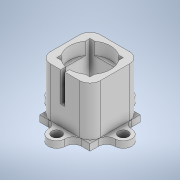
# Autodesk Inventor part: SpringPotBottom
Saved by Autodesk Inventor 2022 (Build 260153000, 153)
## iProperties
Created: 2022-04-06
Part Number: SpringPotBottom
Material: Generic
Document SubType Name: Modeling
Designer: awp
Density: 1 g/cm^3
Appearance: Default
Author: awp
Autodesk Inventor part; units mm, degrees
ref_plane "YZ Plane" through (0, 0, 0) normal (1, 0, 0) x (0, 1, 0)
ref_plane "XZ Plane" through (0, 0, 0) normal (0, 1, 0) x (-1, 0, 0)
ref_plane "XY Plane" through (0, 0, 0) normal (0, 0, 1) x (1, 0, 0)
sketch "Sketch1" plane through (0, 0, 0) normal (0, 1, 0) x (-1, 0, 0)
  line L0 (0, 0) -> (10.125, 0)
  line L1 (10.125, 0) -> (10.125, -10.125)
  line L2 (10.125, -10.125) -> (0, -10.125)
  line L3 (0, -10.125) -> (0, 0)
  line L4 (10.125, -10.125) -> (12.665, -10.125)
  line L5 (12.665, -10.125) -> (12.665, -12.665)
  line L6 (12.665, -12.665) -> (10.125, -12.665)
  line L7 (10.125, -12.665) -> (10.125, -10.125)
  line L8 (0, 0) -> (-2.54, 0)
  line L9 (-2.54, 0) -> (-2.54, 2.54)
  line L10 (-2.54, 2.54) -> (0, 2.54)
  line L11 (0, 2.54) -> (0, 0)
  line L12 (-2.54, 2.54) -> (12.665, 2.54)
  line L13 (12.665, 2.54) -> (12.665, -12.665)
  line L14 (12.665, -12.665) -> (-2.54, -12.665)
  line L15 (-2.54, -12.665) -> (-2.54, 2.54)
  dimension "d0" = 10.125
  dimension "d1" = 10.125
  dimension "d2" = 2.54
  dimension "d3" = 2.54
  dimension "d4" = 2.54
  dimension "d5" = 2.54
  constraints: 32 end point, 8 parallel, 4 horizontal, 4 perpendicular
  measures "d0" distance of L1.end L2.end
  measures "d1" distance of L0.end L1.end
  measures "d2" distance of L5.end L6.end
  measures "d3" distance of L4.end L5.end
  measures "d4" distance of L9.end L10.end
  measures "d5" distance of L8.end L9.end
extrude "Extrusion1" add sketch "Sketch1" along normal blind 8 contours L11 L12 L13 L4 L1 L0 | L3 L2 L7 L14 L15 L8 | L8 L9 L10 L11 | L4 L5 L6 L7
sketch "Sketch2" plane through (0, 8, 0) normal (0, 1, 0) x (1, 0, 0)
  line L0 (2.54, -2.54) -> (-5.0625, -2.54)
  line L1 (-12.665, -2.54) -> (2.54, -2.54) projected
  line L2 (-5.0625, -2.54) -> (-5.0625, 0)
  line L3 (0, 0) -> (-10.125, 0) projected
  line L4 (-5.0625, -2.54) -> (-6.3325, -2.54)
  line L5 (-6.3325, -2.54) -> (-6.3325, 0)
  line L6 (-6.3325, 0) -> (-5.0625, 0)
  line L7 (-12.665, 12.665) -> (-12.665, -2.54) projected
  line L8 (-12.665, -2.54) -> (2.54, -2.54) projected
  line L9 (2.54, -2.54) -> (2.54, 12.665) projected
  line L10 (2.54, 12.665) -> (-12.665, 12.665) projected
  line L11 (-10.125, 10.125) -> (0, 10.125) projected
  line L12 (0, 10.125) -> (0, 0) projected
  line L13 (0, 0) -> (-10.125, 0) projected
  line L14 (-10.125, 0) -> (-10.125, 10.125) projected
  point P0 (-6.3325, 0)
  point P1 (-10.125, 0)
  dimension "d8" = 1.27
  constraints: 10 end point, 2 midpoint, 2 perpendicular, 1 point on line
  measures "d8" distance of L0.end L4.end
extrude "Extrusion2" add sketch "Sketch2" along normal blind 11 contours L0 L2 L3 L12 L11 L14 L5 L1 L7 L10 L9
sketch "Sketch3" plane through (0, 19, 0) normal (0, 1, 0) x (1, 0, 0)
  line L0 (2.54, -2.54) -> (2.54, 12.665) projected
  line L1 (2.54, -2.54) -> (0, 0)
  line L2 (-10.125, 10.125) -> (0, 10.125) projected
  line L3 (2.54, 12.665) -> (0, 10.125)
  line L4 (0, 10.125) -> (0, 0)
  line L5 (2.54, 12.665) -> (-12.665, 12.665) projected
  line L6 (-12.665, -2.54) -> (2.54, -2.54) projected
  line L7 (2.54, 12.665) -> (2.54, -2.54)
  line L8 (-0.8206, 10.125) -> (-0.8206, 12.665)
  line L9 (-10.125, 10.125) -> (-12.665, 12.665)
  line L10 (0, 0) -> (-10.125, 0) projected
  line L11 (-1.9489, 0) -> (-1.1367, -2.54)
  constraints: 14 end point, 4 point on line, 2 perpendicular
extrude "Extrusion3" cut sketch "Sketch3" against normal blind 2
sketch "Sketch4" plane through (0, 19, 0) normal (0, 1, 0) x (1, 0, 0)
  line L0 (-12.665, 12.665) -> (-12.665, -2.54) projected
  line L1 (-12.665, -2.54) -> (-6.3325, -2.54) projected
  line L2 (-6.3325, -2.54) -> (-6.3325, 0) projected
  line L3 (-6.3325, 0) -> (-10.125, 0) projected
  line L4 (-10.125, 0) -> (-10.125, 10.125) projected
  line L5 (-6.3325, 0) -> (-10.125, 0) projected
  line L6 (-5.0625, 0) -> (-5.0625, -2.54) projected
  line L7 (-5.0625, -2.54) -> (-1.1367, -2.54) projected
  line L8 (2.54, 12.665) -> (2.54, -2.54) projected
  line L9 (0, 0) -> (0, 10.125) projected
  line L10 (-12.665, 12.665) -> (-12.665, -2.54) projected
  line L11 (-12.665, 12.665) -> (2.54, 12.665) projected
  line L12 (0, 10.125) -> (-10.125, 10.125) projected
  line L13 (-0.8206, 10.125) -> (-0.8206, 12.665) projected
  line L14 (-0.8206, 10.125) -> (-0.8206, 14.8808)
  line L15 (0, 0) -> (-5.0625, 0) projected
  line L16 (-6.3325, 0) -> (-10.125, 0) projected
  line L17 (-8.3108, 0) -> (-3.1746, 0) construction
  line L18 (-5.0625, 0) -> (-5.0625, -2.54) projected
  line L19 (-5.0625, 0) -> (-2.5225, 0)
  line L20 (-6.3325, 0) -> (-8.8725, 0)
  line L21 (-8.8725, 0) -> (-8.8725, -4.8348)
  line L22 (-2.5225, 0) -> (-2.5225, -5.0399)
  line L23 (-2.5225, 0) -> (2.5174, 0) construction
  circle A0 centre (-5.0625, 5.0625) radius 10.7516
  line L24 (-8.8725, -4.8348) -> (-8.8725, -4.9914)
  line L25 (-2.5225, -5.0399) -> (-2.5225, -5.3847)
  line L26 (-0.8206, 14.8808) -> (-0.8206, 14.9419)
  line L27 (-10.125, 10.125) -> (-12.665, 12.665) projected
  line L28 (-10.125, 10.125) -> (-12.665, 12.665) projected
  line L29 (-6.3325, 0) -> (-6.3325, -3.5818)
  line L30 (-6.3325, 0) -> (-2.7507, 0) construction
  line L31 (-6.3325, -3.5818) -> (-6.3325, -5.6138)
  line L32 (-5.0625, 0) -> (-5.0625, -5.6891)
  line L33 (-5.0625, 0) -> (0.6266, 0) construction
  circle A1 centre (-5.0625, 5.0625) radius 9.525
  line L34 (-1.9489, 0) -> (0, 0) projected
  line L35 (-1.1367, -2.54) -> (-1.9489, 0) projected
  line L36 (2.54, -2.54) -> (-1.1367, -2.54) projected
  line L37 (-1.1367, -2.54) -> (-1.9489, 0) projected
  line L38 (-1.9489, 0) -> (-5.0625, 0) projected
  line L39 (-10.125, 10.125) -> (-12.665, 12.665) projected
  line L40 (-12.665, 12.665) -> (-12.665, -2.54) projected
  line L41 (-12.665, -2.54) -> (-6.3325, -2.54) projected
  line L42 (-6.3325, -2.54) -> (-6.3325, 0) projected
  line L43 (-10.125, 0) -> (-10.125, 10.125) projected
  point P0 (-2.5225, -2.54)
  point P1 (-8.8725, -2.54)
  point P2 (2.54, -0.6758)
  point P3 (-11.7977, 11.7977)
  point P4 (0.6758, -2.54)
  point P5 (2.54, 10.8008)
  point P6 (0.6758, 12.665)
  point P7 (-10.8008, 12.665)
  point P8 (-11.7977, 11.7977)
  point P9 (-5.0625, -4.4625)
  point P10 (-6.3325, -4.3775)
  dimension "d15" = 2.54
  dimension "d16" = 2.54
  dimension "d17" = 90
  dimension "d18" = 90
  dimension "d31" = 90
  dimension "d32" = 90
  dimension "d33" = 19.05
  constraints: 30 end point, 6 point on circle, 4 horizontal, 4 point on line, 3 perpendicular, 2 centre point, 2 vertical, 1 coincident, 1 parallel
  measures "d15" distance of L6.start L19.end
  measures "d16" distance of L2.end L20.end
  measures "d17" angle of L21 L20
  measures "d18" angle of L22 L23
  measures "d31" angle of L29 L30
  measures "d32" angle of L32 L33
  measures "d33" diameter of A1
extrude "Extrusion4" [suppressed]
sketch "Sketch5" plane through (0, 17, 0) normal (0, -1, 0) x (1, 0, 0)
  line L0 (2.54, 0.6758) -> (2.54, 2.54) projected
  arc A0 (2.54, -10.8008) -> (2.54, 0.6758) centre (-5.0625, -5.0625) ccw projected
  line L1 (2.54, -12.665) -> (2.54, -10.8008) projected
  arc A1 (2.54, -12.665) -> (2.54, 2.54) centre (-5.0625, -5.0625) ccw projected
  line L2 (-12.665, 2.54) -> (-12.665, -12.665) projected
  arc A2 (-12.665, 2.54) -> (-12.665, -12.665) centre (-5.0625, -5.0625) ccw projected
  circle A3 centre (-5.0625, -5.0625) radius 10.7516
  circle A4 centre (-5.0625, -5.0625) radius 9.525
  line L3 (-10.8008, -12.665) -> (0.6758, -12.665) projected
  line L4 (2.54, -10.8008) -> (2.54, 0.6758) projected
  line L5 (-5.0625, 4.4625) -> (-5.0625, 2.54) projected
  line L6 (-6.3325, 2.54) -> (-6.3325, 4.3775) projected
  line L7 (-6.3325, 2.54) -> (-12.665, 2.54) projected
  line L8 (-1.1367, 2.54) -> (-5.0625, 2.54) projected
  line L9 (0.6758, 2.54) -> (-1.1367, 2.54) projected
  point P0 (0, 0)
  point P1 (-12.665, -10.8008)
  constraints: 2 centre point, 2 coincident
extrude "Extrusion5" [suppressed]
chamfer "Chamfer4" [suppressed]
chamfer "Chamfer5" [suppressed]
sketch "Sketch6" plane through (0, 0, 0) normal (0, -1, 0) x (1, 0, 0)
  line L0 (-12.665, -12.665) -> (-12.665, 2.54) projected
  line L1 (2.54, -12.665) -> (-12.665, -12.665) projected
  line L2 (2.54, 2.54) -> (2.54, -12.665) projected
  line L3 (-12.665, 2.54) -> (2.54, 2.54) projected
  line L4 (-10.125, -10.125) -> (0, -10.125) projected
  line L5 (-10.125, 0) -> (-10.125, -10.125) projected
  line L6 (0, 0) -> (-10.125, 0) projected
  line L7 (0, -10.125) -> (0, 0) projected
  line L8 (2.54, -12.665) -> (-12.665, -12.665) projected
  line L9 (-5.0625, -12.665) -> (-7.6025, -12.665)
  line L10 (-7.6025, -12.665) -> (-7.6025, -17.745)
  line L11 (-7.6025, -17.745) -> (-5.0625, -17.745)
  line L12 (-5.0625, -17.745) -> (-5.0625, -12.665)
  line L13 (-5.0625, -12.665) -> (-2.5225, -12.665)
  line L14 (-2.5225, -12.665) -> (-2.5225, -17.745)
  line L15 (-2.5225, -17.745) -> (-5.0625, -17.745)
  line L16 (-5.0625, -17.745) -> (-5.0625, -12.665)
  line L17 (-5.0625, 2.54) -> (-7.6025, 2.54)
  line L18 (-7.6025, 2.54) -> (-7.6025, 7.62)
  line L19 (-7.6025, 7.62) -> (-5.0625, 7.62)
  line L20 (-5.0625, 7.62) -> (-5.0625, 2.54)
  line L21 (-12.665, 2.54) -> (2.54, 2.54) projected
  line L22 (-5.0625, 7.62) -> (-2.5225, 7.62)
  line L23 (-2.5225, 7.62) -> (-2.5225, 2.54)
  line L24 (-2.5225, 2.54) -> (-5.0625, 2.54)
  line L25 (-5.0625, 2.54) -> (-5.0625, 7.62)
  circle A0 centre (-5.0625, -15.205) radius 1.5
  circle A1 centre (-5.0625, 5.08) radius 1.5
  line L26 (2.54, 2.54) -> (2.54, -12.665) projected
  line L27 (2.54, -5.0625) -> (7.62, -5.0625)
  line L28 (7.62, -5.0625) -> (7.62, -7.6025)
  line L29 (7.62, -7.6025) -> (2.54, -7.6025)
  line L30 (2.54, -7.6025) -> (2.54, -5.0625)
  line L31 (7.62, -5.0625) -> (2.54, -5.0625)
  line L32 (2.54, -5.0625) -> (2.54, -2.5225)
  line L33 (2.54, -2.5225) -> (7.62, -2.5225)
  line L34 (7.62, -2.5225) -> (7.62, -5.0625)
  line L35 (-12.665, -12.665) -> (-12.665, 2.54) projected
  line L36 (-12.665, -5.0625) -> (-17.745, -5.0625)
  line L37 (-17.745, -5.0625) -> (-17.745, -7.6025)
  line L38 (-17.745, -7.6025) -> (-12.665, -7.6025)
  line L39 (-12.665, -7.6025) -> (-12.665, -5.0625)
  line L40 (-17.745, -5.0625) -> (-12.665, -5.0625)
  line L41 (-12.665, -5.0625) -> (-12.665, -2.5225)
  line L42 (-12.665, -2.5225) -> (-17.745, -2.5225)
  line L43 (-17.745, -2.5225) -> (-17.745, -5.0625)
  circle A2 centre (-15.205, -5.0625) radius 1.5
  circle A3 centre (5.08, -5.0625) radius 1.5
  point P0 (-2.5225, 2.54)
  dimension "d42" = 2.54
  dimension "d43" = 5.08
  dimension "d44" = 2.54
  dimension "d45" = 5.08
  dimension "d46" = 2.54
  dimension "d47" = 3
  dimension "d48" = 2.54
  dimension "d49" = 3
  dimension "d53" = 5.08
  dimension "d54" = 2.54
  dimension "d55" = 2.54
  dimension "d56" = 5.08
  dimension "d57" = 2.54
  dimension "d58" = 2.54
  dimension "d59" = 3
  dimension "d60" = 3
  constraints: 64 end point, 16 parallel, 8 horizontal, 8 midpoint, 8 perpendicular, 4 centre point, 4 point on line
  measures "d42" distance of L11.end L10.end
  measures "d43" distance of L10.end L9.end
  measures "d44" distance of L14.end L15.end
  measures "d45" distance of L17.end L18.end
  measures "d46" distance of L23.end L24.end
  measures "d47" diameter of A0
  measures "d48" distance of L18.end L19.end
  measures "d49" diameter of A1
  measures "d53" distance of L28.end L29.end
  measures "d54" distance of L27.end L28.end
  measures "d55" distance of L31.end L32.end
  measures "d56" distance of L38.end L37.end
  measures "d57" distance of L37.end L36.end
  measures "d58" distance of L41.end L40.end
  measures "d59" diameter of A2
  measures "d60" diameter of A3
extrude "Extrusion6" add sketch "Sketch6" against normal blind 2 contours L38 L37 L36 A2 L0 | L1 L12 A0 L11 L10 | L36 A2 L43 L42 L0 | L1 L14 L15 L12 A0 | L18 L19 L20 A1 L3 | L2 L27 A3 L28 L29 | L20 A1 L22 L23 L3 | L2 L33 L34 L27 A3
fillet "Fillet2" radius 2.54 16 edges at (-7.6025, 1, -17.745) (-2.5225, 1, -17.745) (-2.5225, 1, -12.665) (-7.6025, 1, -12.665) (-7.6025, 1, 2.54) (-2.5225, 1, 2.54) (-2.5225, 1, 7.62) (-7.6025, 1, 7.62) (2.54, 1, -2.5225) (7.62, 1, -2.5225) (7.62, 1, -7.6025) (2.54, 1, -7.6025) (-12.665, 1, -7.6025) (-17.745, 1, -7.6025) (-17.745, 1, -2.5225) (-12.665, 1, -2.5225)
sketch "Sketch7" plane through (-5.0625, 19, -5.0625) normal (0, 1, 0) x (1, 0, 0)
  line L0 (3.9258, -7.6025) -> (3.1136, -5.0625) projected
  line L1 (3.1136, -5.0625) -> (0, -5.0625) projected
  line L2 (0, -5.0625) -> (0, -7.6025) projected
  line L3 (-1.27, -5.0625) -> (-5.0625, -5.0625) projected
  line L4 (-5.0625, -5.0625) -> (-5.0625, 5.0625) projected
  line L5 (-5.0625, 5.0625) -> (-7.6025, 7.6025) projected
  line L6 (-1.27, -5.0625) -> (-5.0625, -5.0625) projected
  line L7 (-1.27, -5.0625) -> (-1.905, -5.0625)
  line L8 (-1.905, -5.0625) -> (-1.905, -9.44)
  line L9 (-1.905, -9.44) -> (-1.27, -9.44)
  line L10 (-1.27, -9.44) -> (-1.27, -5.0625)
  line L11 (-7.6025, 7.6025) -> (-7.6025, -7.6025) projected
  line L12 (-7.6025, -7.6025) -> (-1.27, -7.6025) projected
  line L13 (-1.27, -7.6025) -> (-1.27, -5.0625) projected
  line L14 (0, -7.6025) -> (3.9258, -7.6025) projected
  point P0 (5.0625, -5.0625)
  dimension "d61" = 0.635
  constraints: 8 end point, 2 parallel, 1 horizontal, 1 perpendicular
  measures "d61" distance of L9.end L8.end
extrude "Extrusion7" [suppressed]
fillet "Fillet3" radius 3.175 5 edges at (-12.665, 18, -12.665) (-12.665, 8.5, -12.665) (-12.665, 9.5, 2.54) (2.54, 8.5, 2.54) (2.54, 8.5, -12.665)
sketch "Sketch8" plane through (0, 17, 0) normal (0, 1, 0) x (1, 0, 0)
  arc A0 (2.54, 9.49) -> (-0.635, 12.665) centre (-0.635, 9.49) ccw projected
  line L0 (-9.49, 12.665) -> (-0.635, 12.665) projected
  arc A1 (-9.49, 12.665) -> (-11.7351, 11.7351) centre (-9.49, 9.49) ccw projected
  line L1 (-10.125, 10.125) -> (-11.7351, 11.7351) projected
  line L2 (0, 10.125) -> (-10.125, 10.125) projected
  line L3 (0, 0) -> (0, 10.125) projected
  line L4 (-1.9489, 0) -> (0, 0) projected
  line L5 (-1.1367, -2.54) -> (-1.9489, 0) projected
  line L6 (-0.635, -2.54) -> (-1.1367, -2.54) projected
  arc A2 (-0.635, -2.54) -> (2.54, 0.635) centre (-0.635, 0.635) ccw projected
  line L7 (2.54, 9.49) -> (2.54, 0.635) projected
  arc A3 (-12.665, 0.635) -> (-9.49, -2.54) centre (-9.49, 0.635) ccw projected
  line L8 (-9.49, -2.54) -> (-6.3325, -2.54) projected
  line L9 (-6.3325, -2.54) -> (-6.3325, 0) projected
  line L10 (-6.3325, 0) -> (-10.125, 0) projected
  line L11 (-10.125, 0) -> (-10.125, 10.125) projected
  line L12 (-10.125, 10.125) -> (-11.7351, 11.7351) projected
  arc A4 (-11.7351, 11.7351) -> (-12.665, 9.49) centre (-9.49, 9.49) ccw projected
  line L13 (-12.665, 9.49) -> (-12.665, 0.635) projected
  circle A5 centre (-5.0625, 5.0625) radius 6.25
  point P0 (-1.3973, 0)
  point P1 (-1.8529, -0.3004)
  dimension "d65" = 12.5
  constraints: 1 centre point
  measures "d65" diameter of A5
extrude "Extrusion8" cut sketch "Sketch8" along normal blind 2.54 and the other way blind 3.81 contours A5 L9 L10 L11 L2 L3 L4 L5 | L5 L4 A5 | A5 L2 | L11 A5 | A5 L10 L9 | L3 A5
sketch "Sketch9" plane through (0, 19, 0) normal (0, 1, 0) x (1, 0, 0)
  arc A0 (-8.7277, 0) -> (-6.3325, -1.0571) centre (-5.0625, 5.0625) ccw projected
  line L0 (-8.7277, 0) -> (-10.125, 0) projected
  line L1 (-10.125, 0) -> (-10.125, 1.3973) projected
  arc A1 (-10.125, 8.7277) -> (-10.125, 1.3973) centre (-5.0625, 5.0625) ccw projected
  line L2 (-10.125, 8.7277) -> (-10.125, 10.125) projected
  line L3 (-10.125, 10.125) -> (-11.7351, 11.7351) projected
  arc A2 (-11.7351, 11.7351) -> (-12.665, 9.49) centre (-9.49, 9.49) ccw projected
  line L4 (-12.665, 9.49) -> (-12.665, 0.635) projected
  arc A3 (-12.665, 0.635) -> (-9.49, -2.54) centre (-9.49, 0.635) ccw projected
  line L5 (-9.49, -2.54) -> (-6.3325, -2.54) projected
  line L6 (-6.3325, -2.54) -> (-6.3325, -1.0571) projected
  arc A4 (-5.0625, -1.1875) -> (-1.8529, -0.3004) centre (-5.0625, 5.0625) ccw projected
  line L7 (-5.0625, -1.1875) -> (-5.0625, -2.54) projected
  line L8 (-5.0625, -2.54) -> (-1.1367, -2.54) projected
  line L9 (-1.1367, -2.54) -> (-1.8529, -0.3004) projected
  point P0 (0, 0)
extrude "Extrusion9" cut sketch "Sketch9" against normal up to surface (2 mm away)
body "Solid1"
